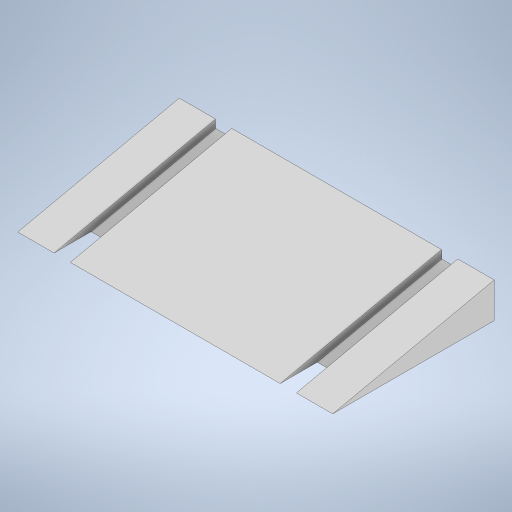
# Autodesk Inventor part: 猫砂盆底座
Saved by Autodesk Inventor 2023.1 (Build 271208000, 208)
## iProperties
Created: 2023-07-19
Part Number: 猫砂盆底座
Material: 常规
Document SubType Name: Modeling
Designer: Selcon
Density: 1 g/cm^3
Appearance: 默认
Author: Selcon
Autodesk Inventor part; units mm, degrees
ref_plane "YZ Plane" through (0, 0, 0) normal (1, 0, 0) x (0, 1, 0)
ref_plane "XZ Plane" through (0, 0, 0) normal (0, 1, 0) x (-1, 0, 0)
ref_plane "XY Plane" through (0, 0, 0) normal (0, 0, 1) x (1, 0, 0)
sketch "草图2" plane through (0, 0, 0) normal (1, 0, 0) x (0, 1, 0)
  line L0 (120, -550) -> (0, 0)
  line L1 (0, 0) -> (0, -550)
  line L2 (0, -550) -> (120, -550)
  line L3 (43.6364, -200) -> (0, -200)
  dimension "d0" = 120
  dimension "d1" = 550
  dimension "d2" = 200
  constraints: 8 end point, 2 perpendicular, 2 point on line, 1 coincident, 1 vertical
  measures "d0" distance of L1.end L0.start
  measures "d1" distance of L0.end L1.end
  measures "d2" distance from line of point (0, 0) L3
extrude "拉伸1" add sketch "草图2" along normal mid plane 390 contours L3 L1 L0
sketch "草图3" plane through (-195, 0, 0) normal (0, 0.9770158, 0.2131671) x (1, 0, 0)
  line L0 (0, 0) -> (390, 0) projected
  line L1 (390, 204.705) -> (0, 204.705) projected
  line L2 (325, 0) -> (345, 0)
  line L3 (345, 0) -> (345, 204.705)
  line L4 (345, 204.705) -> (325, 204.705)
  line L5 (325, 204.705) -> (325, 0)
  line L6 (390, 204.705) -> (390, 0) projected
  point P0 (195, 0)
  dimension "d5" = 20
  dimension "d6" = 45
  constraints: 8 end point, 2 parallel, 2 point on line, 1 horizontal, 1 perpendicular
  measures "d5" distance between parallel lines of L3 L5
  measures "d6" distance between parallel lines of L6 L3
sketch "草图4" plane through (195, 43.6364, -200) normal (0, 0, -1) x (-1, 0, 0)
  line L0 (45, 0) -> (45, -10)
  point P0 (195, -43.6364)
  dimension "d8" = 10
  constraints: 2 end point, 1 vertical
  measures "d8" distance of L0.start L0.end
sweep "扫掠1" cut profiles "草图3" path "草图4" contours L5 L1 L3 L0
mirror "镜像1" about plane through (0, 0, 0) normal (1, 0, 0) of "扫掠1"
sketch "草图5" plane through (-195, 0, -200) normal (0, -1, 0) x (1, 0, 0)
  line L0 (195, -50) -> (195, 300) projected
  line L1 (0, 0) -> (390, 0) projected
  line L2 (210, 0) -> (180, 0)
  line L3 (180, 0) -> (180, 60)
  line L4 (180, 60) -> (210, 60)
  line L5 (210, 60) -> (210, 0)
  point P0 (195, 200)
  point P1 (180, 0)
  dimension "d11" = 60
  dimension "d12" = 30
  constraints: 8 end point, 2 parallel, 1 horizontal, 1 perpendicular, 1 point on line, 1 other
  measures "d11" distance of L2.end L3.end
  measures "d12" distance between parallel lines of L3 L5
extrude "拉伸2" cut sketch "草图5" against normal blind 15
sketch "草图6" plane through (-195, 15, -200) normal (0, -1, 0) x (1, 0, 0)
  line L0 (210, 0) -> (180, 0) projected
  line L1 (180, 60) -> (210, 60) projected
  line L2 (180, 0) -> (180, 60) projected
  line L3 (210, 0) -> (180, 0) projected
  line L4 (210, 60) -> (210, 0) projected
  line L5 (195, -11.4626) -> (195, 50.2539)
  circle A0 centre (195, 25) radius 6
  circle A1 centre (195, 45) radius 6
  point P0 (195, 200)
  dimension "d15" = 30
  dimension "d16" = 12
  dimension "d17" = 12
  dimension "d18" = 20
  dimension "d19" = 25
  constraints: 2 centre point, 2 end point, 2 point on line, 1 vertical
  measures "d15" diameter of L2 L5
  measures "d16" diameter of A0
  measures "d17" diameter of A1
  measures "d18" distance of A0.centre A1.centre
  measures "d19" distance from line of L0 A0.centre
extrude "拉伸3" cut sketch "草图6" against normal blind 15 contours A0 L5 | L5 A0 | A1
thread "螺纹1"
thread "螺纹2"
